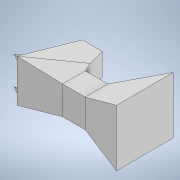
# Autodesk Inventor part: horse
Saved by Autodesk Inventor 2021 (Build 250183000, 183)
## iProperties
Created: 2021-01-20
Part Number: horse
Material: Generic
Document SubType Name: Modeling
Designer: Luke Kamols
Density: 1 g/cm^3
Appearance: Default
Author: Luke Kamols
Autodesk Inventor part; units mm, degrees
sketch "Sketch1" plane through (0, 0, 0) normal (0, 1, 0) x (-1, 0, 0)
  line L0 (0, 0) -> (40, 0)
  line L1 (0, 0) -> (0, -20)
  line L2 (0, 0) -> (0, -10)
  line L3 (37, -20) -> (40, 0)
  line L4 (37, -20) -> (30, -20)
  line L5 (26, -10) -> (30, -20)
  line L6 (26, -10) -> (18, -10)
  line L7 (0, -20) -> (5, -20)
  line L8 (5, -20) -> (18, -10)
  line L9 (18, 0) -> (18, -2)
  line L10 (18, -2) -> (5, 0)
  line L11 (18, -2) -> (26, -2)
  line L12 (26, -2) -> (40, 0)
  dimension "d1" = 40
  dimension "d2" = 20
  dimension "d7" = 10
  dimension "d8" = 37
  dimension "d9" = 7
  dimension "d10" = 26
  dimension "d11" = 8
  dimension "d12" = 5
  dimension "d33" = 2
  constraints: 26 end point, 4 horizontal, 2 point on line, 2 vertical, 1 midpoint
  measures "d1" distance of L0.start L0.end
  measures "d2" distance of L0.start L1.end
  measures "d7" distance of L0.start L2.end
  measures "d8" distance of L1.end L3.start
  measures "d9" distance of L3.start L4.end
  measures "d10" distance of L2.end L5.start
  measures "d11" distance of L5.start L6.end
  measures "d12" distance of L1.end L7.end
  measures "d33" distance of L9.start L9.end
extrude "Extrusion1" add sketch "Sketch1" along normal blind 20 contours L0 L10 L11 L12 L3 L4 L5 L6 L8 L7 L1
sketch "Sketch2" plane through (-40, 0, 0) normal (0, 0, 1) x (1, 0, 0)
  line L0 (3, 0) -> (3, 20) projected
  line L1 (10, 0) -> (10, 20) projected
  line L2 (14, 0) -> (14, 20) projected
  line L3 (22, 0) -> (22, 20) projected
  line L4 (35, 0) -> (35, 20) projected
  line L5 (40, 0) -> (40, 20) projected
  line L6 (0, 0) -> (0, 20) projected
  line L7 (0, 20) -> (40, 20) projected
  line L8 (35, 0) -> (40, 0) projected
  line L9 (40, 0) -> (40, 20) projected
  line L10 (35, 20) -> (40, 20) projected
  line L11 (40, 0) -> (40, 20) projected
  line L12 (40, 10) -> (0, 10)
  line L13 (22, 0) -> (22, 5)
  line L14 (35, 0) -> (22, 0) projected
  line L15 (22, 5) -> (35, 0)
  line L16 (22, 5) -> (14, 5)
  line L17 (10, 0) -> (10, 2.5)
  line L18 (10, 2.5) -> (14, 5)
  line L19 (10, 2.5) -> (3, 2.5)
  line L20 (22, 15) -> (35, 20)
  line L21 (22, 15) -> (14, 15)
  line L22 (10, 17.5) -> (14, 15)
  line L23 (10, 17.5) -> (3, 17.5)
  line L24 (3, 17.5) -> (0, 17.5)
  line L25 (3, 2.5) -> (0, 2.5)
  line L26 (14, 5) -> (0, 2.5)
  line L27 (14, 15) -> (0, 17.5)
  line L28 (35, 0) -> (35, 20) projected
  line L29 (0, 0) -> (14, 0) projected
  line L30 (0, 0) -> (40, 0)
  dimension "d15" = 5
  dimension "d16" = 2.5
  constraints: 32 end point, 5 point on line, 4 symmetric about line, 3 perpendicular, 1 horizontal, 1 midpoint
  measures "d15" distance of L3.start L13.end
  measures "d16" distance of L1.start L17.end
extrude "Extrusion2" cut sketch "Sketch2" against normal blind 20 contours L29 L6 L25 L0 | L0 L19 L1 L29 | L25 L26 L0 | L0 L26 L1 L19 | L1 L18 L2 L29 | L1 L26 L18 | L2 L16 L3 L30 | L3 L15 L14 | L27 L24 L0 | L0 L23 L1 L27 | L6 L7 L0 L24 | L4 L12 L5 L8 | L0 L7 L1 L23 | L1 L22 L27 | L22 L1 L7 L2 | L2 L7 L3 L21 | L4 L7 L5 L12 | L3 L7 L20
ref_plane "Work Plane1" through (-40, 0, 0) normal (1, 0, 0) x (0, 0, -1)
sketch "Sketch4" plane through (-40, 0, 0) normal (1, 0, 0) x (0, 0, -1)
  line L0 (0, 17.5) -> (20, 16.9643) projected
  line L1 (20, 3.0357) -> (20, 16.9643) projected
  line L2 (20, 3.0357) -> (0, 2.5) projected
  line L3 (20, 3.0357) -> (20, 16.9643) projected
  line L4 (20, 3.0357) -> (20, 6.0357)
  line L5 (20, 16.9643) -> (20, 13.9643)
  line L6 (20, 4.2857) -> (20, 15.7143) projected
  line L7 (0, 2.5) -> (0, 17.5) projected
  line L8 (0, 2.5) -> (20, 6.0357)
  line L9 (0, 17.5) -> (20, 16.9643) projected
  line L10 (20, 13.9643) -> (0, 17.5)
  point P0 (0, 0)
  dimension "d24" = 3
  dimension "d25" = 3
  constraints: 8 end point, 2 point on line
  measures "d24" distance of L1.start L4.end
  measures "d25" distance of L0.end L5.end
extrude "Extrusion4" cut sketch "Sketch4" along normal blind 22 contours L0 L1 L10 | L8 L1 L2
sketch "Sketch5" plane through (-40, 2.5, 0) normal (-0.9889364, 0, -0.1483405) x (-0.1483405, 0, 0.9889364)
  line L0 (0, 0) -> (0, 15) projected
  line L1 (0, 14) -> (-1, 14)
  line L2 (-4.0546, 12.5) -> (-11.9661, 12.5) projected
  line L3 (-5.5, 12.5) -> (-1, 14)
  line L4 (0, 11) -> (-1, 11)
  line L5 (-1, 14) -> (-1, 11)
  line L6 (-5.5, 12.5) -> (-1, 11)
  point P0 (-5.9336, -2.5)
  point P1 (-4.8339, 12.5)
  dimension "d53" = 1
  dimension "d55" = 1
  constraints: 10 end point, 1 horizontal, 1 perpendicular, 1 point on line, 1 vertical
  measures "d53" distance of L1.start L1.end
  measures "d55" distance of L4.start L4.end
ref_plane "Work Plane3" through (-43.9557, 2.5, -0.5934) normal (-0.9889364, 0, -0.1483405) x (-0.1483405, 0, 0.9889364)
sketch "Sketch8" plane through (-43.9557, 2.5, -0.5934) normal (-0.9889364, 0, -0.1483405) x (-0.1483405, 0, 0.9889364)
  line L0 (-5.5, 12.5) -> (-1, 14) projected
  line L1 (-1, 14) -> (-1, 11) projected
  line L2 (-5.5, 12.5) -> (-1, 11) projected
  line L3 (-1, 12.5) -> (-2, 12.5)
  point P0 (-5.9336, -2.5)
  dimension "d56" = 1
  constraints: 2 end point, 1 coincident, 1 horizontal, 1 midpoint
  measures "d56" distance of L3.start L3.end
loft "Loft3" add profiles "Sketch5" section 1 point at (-43.6591, 15, -2.5712) contours L6 L3 L5
ref_plane "Work Plane4" through (-37, 10, -42.4242) normal (0, 1, 0) x (1, 0, 0)
mirror "Mirror1" about plane through (-37, 10, -42.4242) normal (0, 1, 0) of "Loft3"
body "Solid1"
